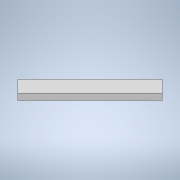
# Autodesk Inventor part: examplePart
Saved by Autodesk Inventor 2020.2 (Build 242310000, 310)
## iProperties
Created: 2020-02-12
Part Number: examplePart
Material: Generic
Document SubType Name: Modeling
Designer: robst
Density: 1 g/cm^3
Appearance: Default
Author: robst
Autodesk Inventor part; units mm, degrees
ref_plane "YZ Plane" through (0, 0, 0) normal (1, 0, 0) x (0, 1, 0)
ref_plane "XZ Plane" through (0, 0, 0) normal (0, 1, 0) x (-1, 0, 0)
ref_plane "XY Plane" through (0, 0, 0) normal (0, 0, 1) x (1, 0, 0)
sketch "Sketch1" plane through (0, 0, 0) normal (0, 1, 0) x (-1, 0, 0)
  line L0 (44.9013, 62.8618) -> (-62.8618, -44.9013)
  line L1 (-62.8618, -44.9013) -> (-44.9013, -62.8618)
  line L2 (-44.9013, -62.8618) -> (62.8618, 44.9013)
  line L3 (62.8618, 44.9013) -> (44.9013, 62.8618)
  line L4 (44.9013, 62.8618) -> (-44.9013, -62.8618) construction
  line L5 (-62.8618, -44.9013) -> (62.8618, 44.9013) construction
  line L6 (44.9013, 62.8618) -> (197.3013, 62.8618) construction
  point P0 (0, 0)
  dimension "d0" = 152.4
  dimension "d1" = 135
  dimension "d2" = 25.4
  constraints: 14 end point, 2 midpoint, 2 parallel, 1 equal length, 1 horizontal, 1 perpendicular
  measures "d0" distance of L0.start L0.end
  measures "d1" angle of L0 L6
  measures "d2" distance of L1.end L0.end
extrude "Extrusion1" add sketch "Sketch1" along normal mid plane 9.525
body "Solid1"
